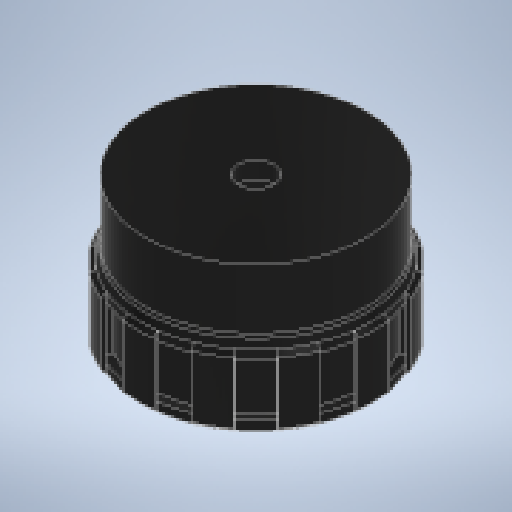
# Autodesk Inventor part: Motor Hub
Saved by Autodesk Inventor 2023.2 (Build 272271000, 271)
## iProperties
Created: 2022-12-29
Part Number: Motor Hub
Material: Nylon 6/6
Document SubType Name: Modeling
Designer: Nathan Cai
Density: 1.13 g/cm^3
Appearance: Smooth - Black
Mass: 9.71742 g
Surface Area: 89.0077 cm^2
Volume: 8.59949 cm^3
Author: Nathan Cai
Autodesk Inventor part; units mm, degrees
ref_plane "YZ Plane" through (0, 0, 0) normal (1, 0, 0) x (0, 1, 0)
ref_plane "XZ Plane" through (0, 0, 0) normal (0, 1, 0) x (-1, 0, 0)
ref_plane "XY Plane" through (0, 0, 0) normal (0, 0, 1) x (1, 0, 0)
sketch "Sketch1" plane through (0, 0, 0) normal (0, 1, 0) x (-1, 0, 0)
  circle A0 centre (0, 0) radius 22.225 construction
  circle A1 centre (0, 0) radius 17.6
  circle A2 centre (0, 0) radius 19.05
  dimension "d0" = 44.45
  dimension "d1" = 35.2
  dimension "d2" = 38.1
  constraints: 3 centre point, 3 coincident
  measures "d0" diameter of A0
  measures "d1" diameter of A1
  measures "d2" diameter of A2
extrude "Extrusion1" add sketch "Sketch1" along normal blind 9.525
sketch "Sketch2" plane through (0, 0, 0) normal (0, -1, 0) x (1, 0, 0)
  circle A0 centre (0, 0) radius 17.6
  circle A1 centre (0, 0) radius 20.6375
  dimension "d5" = 41.275
  dimension "d6" = 35.2
  constraints: 2 centre point, 2 coincident
  measures "d5" diameter of A1
  measures "d6" diameter of A0
extrude "Extrusion2" add sketch "Sketch2" along normal blind 1.5875
sketch "Sketch3" plane through (0, 9.525, 0) normal (0, 1, 0) x (1, 0, 0)
  circle A0 centre (0, 0) radius 17.6
  circle A1 centre (0, 0) radius 20.6375
  dimension "d9" = 35.2
  dimension "d10" = 41.275
  constraints: 2 centre point, 2 coincident
  measures "d9" diameter of A0
  measures "d10" diameter of A1
extrude "Extrusion3" add sketch "Sketch3" along normal blind 1.5875
sketch "Sketch4" plane through (0, 0, 0) normal (1, 0, 0) x (0, 1, 0)
  line L0 (11.1125, -17.6) -> (17.8875, -17.6)
  line L1 (17.8875, -17.6) -> (17.8875, -20.6375)
  line L2 (17.8875, -20.6375) -> (11.1125, -20.6375) construction
  line L3 (11.1125, -20.6375) -> (11.1125, -17.6)
  line L4 (11.1125, -20.6375) -> (11.1125, 20.6375) projected
  line L5 (12.7, -17.6) -> (12.7, -20.6375) construction
  line L6 (11.1125, -20.6375) -> (12.7, -19.8438)
  line L7 (12.7, -19.8438) -> (17.8875, -19.8438)
  line L8 (0, 0) -> (25.7056, 0) construction
  line L9 (-11.1125, 0) -> (-11.1125, -19.8438) construction
  line L10 (0, 20.6375) -> (0, -20.6375) projected
  dimension "d13" = 17.6
  dimension "d14" = 20.6375
  dimension "d16" = 1.5875
  dimension "d18" = 19.8438
  dimension "d84" = 11.1125
  dimension "d85" = 29
  constraints: 18 end point, 5 point on line, 3 parallel, 2 horizontal, 2 perpendicular, 1 vertical
  measures "d13" distance from line of L8.start L0
  measures "d14" distance from line of L8.start L2
  measures "d16" distance between parallel lines of L3 L5
  measures "d18" vertical distance of L8.start L7.end
  measures "d84" distance between parallel lines of L9 L10
  measures "d85" distance between parallel lines of L9 L1
revolve "Revolution1" add sketch "Sketch4" angle 360 about axis through (0, 0, 0) along (0, 1, 0)
sketch "Sketch8" plane through (0, 0, 0) normal (0, 1, 0) x (1, 0, 0)
  circle A0 centre (0, 0) radius 19.05
  circle A1 centre (0, 0) radius 20.6375
  circle A2 centre (0, 0) radius 19.05 projected
  line L0 (0, 0) -> (0, 20.6375) construction
  circle A3 centre (0, 0) radius 20.6375 projected
  line L1 (-0.7937, 18.241) -> (0.7938, 18.241)
  line L2 (0.7938, 18.241) -> (0.7937, 20.6222)
  line L3 (0.7937, 20.6222) -> (-0.7937, 20.6222) construction
  line L4 (-0.7937, 20.6222) -> (-0.7937, 18.241)
  line L5 (-0.7937, 18.241) -> (0.7937, 20.6222) construction
  line L6 (0.7938, 18.241) -> (-0.7937, 20.6222) construction
  line L7 (-9.8079, 15.4003) -> (-8.4331, 16.194)
  line L8 (-8.4331, 16.194) -> (-9.6237, 18.2563)
  line L9 (-9.6237, 18.2563) -> (-10.9985, 17.4625) construction
  line L10 (-10.9985, 17.4625) -> (-9.8079, 15.4003)
  line L11 (-9.8079, 15.4003) -> (-9.6237, 18.2563) construction
  line L12 (-8.4331, 16.194) -> (-10.9985, 17.4625) construction
  line L13 (-16.194, 8.4331) -> (-15.4003, 9.8079)
  line L14 (-15.4003, 9.8079) -> (-17.4625, 10.9985)
  line L15 (-17.4625, 10.9985) -> (-18.2563, 9.6237) construction
  line L16 (-18.2563, 9.6237) -> (-16.194, 8.4331)
  line L17 (-16.194, 8.4331) -> (-17.4625, 10.9985) construction
  line L18 (-15.4003, 9.8079) -> (-18.2563, 9.6237) construction
  line L19 (-18.241, -0.7937) -> (-18.241, 0.7938)
  line L20 (-18.241, 0.7938) -> (-20.6222, 0.7938)
  line L21 (-20.6222, 0.7938) -> (-20.6222, -0.7937) construction
  line L22 (-20.6222, -0.7937) -> (-18.241, -0.7937)
  line L23 (-18.241, -0.7937) -> (-20.6222, 0.7938) construction
  line L24 (-18.241, 0.7938) -> (-20.6222, -0.7937) construction
  line L25 (-15.4003, -9.8079) -> (-16.194, -8.4331)
  line L26 (-16.194, -8.4331) -> (-18.2563, -9.6237)
  line L27 (-18.2563, -9.6237) -> (-17.4625, -10.9985) construction
  line L28 (-17.4625, -10.9985) -> (-15.4003, -9.8079)
  line L29 (-15.4003, -9.8079) -> (-18.2563, -9.6237) construction
  line L30 (-16.194, -8.4331) -> (-17.4625, -10.9985) construction
  line L31 (-8.4331, -16.194) -> (-9.8079, -15.4003)
  line L32 (-9.8079, -15.4003) -> (-10.9985, -17.4625)
  line L33 (-10.9985, -17.4625) -> (-9.6237, -18.2563) construction
  line L34 (-9.6237, -18.2563) -> (-8.4331, -16.194)
  line L35 (-8.4331, -16.194) -> (-10.9985, -17.4625) construction
  line L36 (-9.8079, -15.4003) -> (-9.6237, -18.2563) construction
  line L37 (0.7937, -18.241) -> (-0.7938, -18.241)
  line L38 (-0.7938, -18.241) -> (-0.7938, -20.6222)
  line L39 (-0.7938, -20.6222) -> (0.7937, -20.6222) construction
  line L40 (0.7937, -20.6222) -> (0.7937, -18.241)
  line L41 (0.7937, -18.241) -> (-0.7938, -20.6222) construction
  line L42 (-0.7938, -18.241) -> (0.7937, -20.6222) construction
  line L43 (9.8079, -15.4003) -> (8.4331, -16.194)
  line L44 (8.4331, -16.194) -> (9.6237, -18.2563)
  line L45 (9.6237, -18.2563) -> (10.9985, -17.4625) construction
  line L46 (10.9985, -17.4625) -> (9.8079, -15.4003)
  line L47 (9.8079, -15.4003) -> (9.6237, -18.2563) construction
  line L48 (8.4331, -16.194) -> (10.9985, -17.4625) construction
  line L49 (16.194, -8.4331) -> (15.4003, -9.8079)
  line L50 (15.4003, -9.8079) -> (17.4625, -10.9985)
  line L51 (17.4625, -10.9985) -> (18.2563, -9.6237) construction
  line L52 (18.2563, -9.6237) -> (16.194, -8.4331)
  line L53 (16.194, -8.4331) -> (17.4625, -10.9985) construction
  line L54 (15.4003, -9.8079) -> (18.2563, -9.6237) construction
  line L55 (18.241, 0.7937) -> (18.241, -0.7938)
  line L56 (18.241, -0.7938) -> (20.6222, -0.7938)
  line L57 (20.6222, -0.7938) -> (20.6222, 0.7937) construction
  line L58 (20.6222, 0.7937) -> (18.241, 0.7937)
  line L59 (18.241, 0.7937) -> (20.6222, -0.7938) construction
  line L60 (18.241, -0.7938) -> (20.6222, 0.7937) construction
  line L61 (15.4003, 9.8079) -> (16.194, 8.4331)
  line L62 (16.194, 8.4331) -> (18.2563, 9.6237)
  line L63 (18.2563, 9.6237) -> (17.4625, 10.9985) construction
  line L64 (17.4625, 10.9985) -> (15.4003, 9.8079)
  line L65 (15.4003, 9.8079) -> (18.2563, 9.6237) construction
  line L66 (16.194, 8.4331) -> (17.4625, 10.9985) construction
  line L67 (8.4331, 16.194) -> (9.8079, 15.4003)
  line L68 (9.8079, 15.4003) -> (10.9985, 17.4625)
  line L69 (10.9985, 17.4625) -> (9.6237, 18.2562) construction
  line L70 (9.6237, 18.2562) -> (8.4331, 16.194)
  line L71 (8.4331, 16.194) -> (10.9985, 17.4625) construction
  line L72 (9.8079, 15.4003) -> (9.6237, 18.2562) construction
  point P0 (0, 19.4316)
  point P1 (-10.3187, 17.8726)
  point P2 (-9.7158, 16.8283)
  point P3 (-17.8726, 10.3188)
  point P4 (-16.8283, 9.7158)
  point P5 (-20.6375, 0)
  point P6 (-19.4316, 0)
  point P7 (-17.8726, -10.3187)
  point P8 (-16.8283, -9.7158)
  point P9 (-10.3188, -17.8726)
  point P10 (-9.7158, -16.8283)
  point P11 (0, -20.6375)
  point P12 (0, -19.4316)
  point P13 (10.3187, -17.8726)
  point P14 (9.7158, -16.8283)
  point P15 (17.8726, -10.3188)
  point P16 (16.8283, -9.7158)
  point P17 (20.6375, 0)
  point P18 (19.4316, 0)
  point P19 (17.8726, 10.3187)
  point P20 (16.8283, 9.7158)
  point P21 (10.3188, 17.8726)
  point P22 (9.7158, 16.8283)
  point P23 (16.0866, 10.2041)
  point P24 (16.8803, 8.8293)
  point P25 (19.0335, 0.7937)
  point P26 (19.0335, -0.7938)
  point P27 (16.8803, -8.8293)
  point P28 (16.0866, -10.2041)
  point P29 (10.2041, -16.0866)
  point P30 (8.8293, -16.8803)
  point P31 (0.7937, -19.0335)
  point P32 (-0.7938, -19.0335)
  point P33 (-16.0866, -10.2041)
  point P34 (-16.8803, -8.8293)
  point P35 (-8.8293, -16.8803)
  point P36 (-10.2041, -16.0866)
  point P37 (-19.0335, -0.7937)
  point P38 (-19.0335, 0.7938)
  point P39 (-16.8803, 8.8293)
  point P40 (-16.0866, 10.2041)
  point P41 (-10.2041, 16.0866)
  point P42 (-8.8293, 16.8803)
  point P43 (-0.7937, 19.0335)
  point P44 (0.7938, 19.0335)
  point P45 (8.8293, 16.8803)
  point P46 (10.2041, 16.0866)
  dimension "d67" = 41.275
  dimension "d68" = 38.1
  dimension "d77" = 1.5875
  dimension "d78" = 2.3813
  dimension "d81" = 360
  constraints: 146 end point, 2 coincident, 2 midpoint, 2 parallel, 2 point on circle, 1 horizontal, 1 perpendicular, 1 point on line, 1 vertical, 149 other
  measures "d77" distance of L3.end L2.end
  measures "d78" distance between parallel lines of L3 L1
extrude "Extrusion7" add sketch "Sketch8" along normal blind 9.525 contours A0 L58 A1 L56 | A0 L64 A1 L62 | L52 A1 L50 A0 | A0 L70 A1 L68 | L46 A1 L44 A0 | A0 L4 A1 L2 | L40 A1 L38 A0 | A0 L10 A1 L8 | L34 A1 L32 A0 | A0 L16 A1 L14 | L28 A1 L26 A0 | A0 L22 A1 L20
fillet "Fillet4" radius 1.5875 1 edges at (0, 12.7, 19.8438)
ref_plane "Work Plane1" through (0, 4.7625, 0) normal (0, 1, 0) x (1, 0, 0)
sketch "Sketch10" plane through (0, 4.7625, 0) normal (0, 1, 0) x (1, 0, 0)
  circle A0 centre (0, 0) radius 21.4312
  circle A1 centre (0, 0) radius 20.6375
  line L0 (0, 0) -> (2.7973, 21.2479)
  line L1 (0, 0) -> (0, 21.4312) construction
  line L2 (0, 0) -> (-2.7973, 21.2479)
  line L3 (0, 0) -> (-8.2014, 19.7999)
  line L4 (0, 0) -> (-13.0465, 17.0026)
  line L5 (0, 0) -> (-17.0026, 13.0465)
  line L6 (0, 0) -> (-19.7999, 8.2014)
  line L7 (0, 0) -> (-21.2479, 2.7973)
  line L8 (0, 0) -> (-21.2479, -2.7973)
  line L9 (0, 0) -> (-19.7999, -8.2014)
  line L10 (0, 0) -> (-17.0026, -13.0465)
  line L11 (0, 0) -> (-13.0465, -17.0026)
  line L12 (0, 0) -> (-8.2014, -19.7999)
  line L13 (0, 0) -> (-2.7973, -21.2479)
  line L14 (0, 0) -> (2.7973, -21.2479)
  line L15 (0, 0) -> (8.2014, -19.7999)
  line L16 (0, 0) -> (13.0465, -17.0026)
  line L17 (0, 0) -> (17.0026, -13.0465)
  line L18 (0, 0) -> (19.7999, -8.2014)
  line L19 (0, 0) -> (21.2479, -2.7973)
  line L20 (0, 0) -> (21.2479, 2.7973)
  line L21 (0, 0) -> (19.7999, 8.2014)
  line L22 (0, 0) -> (17.0026, 13.0465)
  line L23 (0, 0) -> (13.0465, 17.0026)
  line L24 (0, 0) -> (8.2014, 19.7999)
  point P0 (-2.6937, 20.4609)
  point P1 (2.6937, 20.4609)
  point P2 (-12.5633, 16.3728)
  point P3 (-7.8976, 19.0666)
  point P4 (-19.0666, 7.8976)
  point P5 (-16.3728, 12.5633)
  point P6 (-20.4609, -2.6937)
  point P7 (-20.4609, 2.6937)
  point P8 (-16.3728, -12.5633)
  point P9 (-19.0666, -7.8976)
  point P10 (-7.8976, -19.0666)
  point P11 (-12.5633, -16.3728)
  point P12 (2.6937, -20.4609)
  point P13 (-2.6937, -20.4609)
  point P14 (12.5633, -16.3728)
  point P15 (7.8976, -19.0666)
  point P16 (19.0666, -7.8976)
  point P17 (16.3728, -12.5633)
  point P18 (20.4609, 2.6937)
  point P19 (20.4609, -2.6937)
  point P20 (16.3728, 12.5633)
  point P21 (19.0666, 7.8976)
  point P22 (7.8976, 19.0666)
  point P23 (12.5633, 16.3728)
  dimension "d109" = 42.8625
  dimension "d110" = 41.275
  dimension "d113" = 7.5
  dimension "d116" = 360
  constraints: 50 end point, 2 coincident, 1 symmetric about line, 1 vertical, 67 other
  measures "d113" angle of L1 L0
extrude "Extrusion9" add sketch "Sketch10" along normal mid plane 12.7 contours A0 L19 A1 L20 | L21 A1 L22 A0 | A0 L17 A1 L18 | L23 A1 L24 A0 | A1 L2 A0 L0 | A1 L4 A0 L3 | A1 L6 A0 L5 | A1 L8 A0 L7 | A1 L10 A0 L9 | A1 L12 A0 L11 | A1 L14 A0 L13 | A1 L16 A0 L15
chamfer "Chamfer4" distance 0.7937 angle 45 25 edges at (0, 11.1125, 21.4312) (10.7156, 11.1125, 18.56) (18.56, 11.1125, 10.7156) (21.4312, 11.1125, 0) (18.56, 11.1125, -10.7156) (10.7156, 11.1125, -18.56) (18.56, -1.5875, -10.7156) (21.4312, -1.5875, 0) (18.56, -1.5875, 10.7156) (10.7156, -1.5875, 18.56) (0, -1.5875, 21.4312) (-10.7156, -1.5875, 18.56) (0, 11.1125, -21.4312) (-10.7156, 11.1125, -18.56) (-18.56, 11.1125, -10.7156) (-21.4312, 11.1125, 0) (-18.56, 11.1125, 10.7156) (-10.7156, 11.1125, 18.56) (10.7156, -1.5875, -18.56) (8.0495, 11.1125, -19.4332) (0, -1.5875, -21.4312) (-10.7156, -1.5875, -18.56) (-18.56, -1.5875, -10.7156) (-21.4312, -1.5875, 0) (-18.56, -1.5875, 10.7156)
sketch "Sketch11" plane through (0, 17.8875, 0) normal (0, 1, 0) x (1, 0, 0)
  circle A0 centre (0, 0) radius 11.75 construction
  line L0 (0, 0) -> (-11.75, 0) construction
  circle A1 centre (-11.75, 0) radius 3.875
  line L1 (-11.75, -3.875) -> (-18.1, -3.875)
  line L2 (-18.1, -3.875) -> (-18.1, 3.875)
  line L3 (-18.1, 3.875) -> (-11.75, 3.875)
  line L4 (-11.75, 3.875) -> (-11.75, -3.875) construction
  circle A2 centre (0, -11.75) radius 3.875
  line L5 (3.875, -11.75) -> (3.875, -18.1)
  line L6 (3.875, -18.1) -> (-3.875, -18.1)
  line L7 (-3.875, -18.1) -> (-3.875, -11.75)
  line L8 (-3.875, -11.75) -> (3.875, -11.75) construction
  circle A3 centre (11.75, 0) radius 3.875
  line L9 (11.75, 3.875) -> (18.1, 3.875)
  line L10 (18.1, 3.875) -> (18.1, -3.875)
  line L11 (18.1, -3.875) -> (11.75, -3.875)
  line L12 (11.75, -3.875) -> (11.75, 3.875) construction
  circle A4 centre (0, 11.75) radius 3.875
  line L13 (-3.875, 11.75) -> (-3.875, 18.1)
  line L14 (-3.875, 18.1) -> (3.875, 18.1)
  line L15 (3.875, 18.1) -> (3.875, 11.75)
  line L16 (3.875, 11.75) -> (-3.875, 11.75) construction
  point P0 (3.875, 11.75)
  point P1 (11.75, -3.875)
  point P2 (-3.875, -11.75)
  point P3 (-11.75, 3.875)
  dimension "d121" = 23.5
  dimension "d122" = 7.75
  dimension "d123" = 6.35
  dimension "d126" = 360
  constraints: 34 end point, 5 coincident, 4 horizontal, 2 parallel, 1 horizontal alignment, 1 perpendicular, 59 other
  measures "d123" distance of L2.end L3.end
extrude "Extrusion10" add sketch "Sketch11" against normal blind 3
fillet "Fillet5" radius 0.5 8 edges at (-17.1681, 16.3875, -3.875) (-17.1681, 16.3875, 3.875) (-3.875, 16.3875, 17.1681) (3.875, 16.3875, 17.1681) (17.1681, 16.3875, -3.875) (17.1681, 16.3875, 3.875) (-3.875, 16.3875, -17.1681) (3.875, 16.3875, -17.1681)
chamfer "Chamfer5" distance 1.5875 angle 45 1 edges at (-17.6, -1.5875, 0)
body "Solid1"
